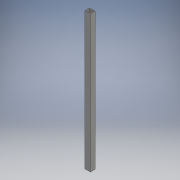
# Autodesk Inventor part: perfil aluminio
Saved by Autodesk Inventor 2016 (Build 200138000, 138)
## iProperties
Created: 2016-06-24
Part Number: perfil aluminio
Material: Generic
Document SubType Name: Modeling
Designer: Admin
Density: 1 g/cm^3
Appearance: Default
Author: Admin
Autodesk Inventor part; units mm, degrees
ref_plane "YZ Plane" through (0, 0, 0) normal (1, 0, 0) x (0, 1, 0)
ref_plane "XZ Plane" through (0, 0, 0) normal (0, 1, 0) x (-1, 0, 0)
ref_plane "XY Plane" through (0, 0, 0) normal (0, 0, 1) x (1, 0, 0)
sketch "Sketch1" plane through (0, 0, 0) normal (0, 0, 1) x (1, 0, 0)
  line L0 (0, 0) -> (12, 0)
  line L1 (12, 0) -> (12, 10)
  line L2 (12, 10) -> (0, 10)
  line L3 (0, 10) -> (0, 0)
  dimension "d0" = 12
  dimension "d1" = 10
  constraints: 8 end point, 2 parallel, 1 horizontal, 1 perpendicular
  measures "d0" distance of L2.end L1.end
  measures "d1" distance of L1.end L0.end
extrude "Extrusion1" add sketch "Sketch1" along normal blind 300
sketch "Sketch3" plane through (0, 0, 300) normal (0, 0, 1) x (1, 0, 0)
  line L0 (12, 10) -> (0, 10) projected
  line L1 (1, 1) -> (11, 1)
  line L2 (11, 1) -> (11, 9)
  line L3 (11, 9) -> (1, 9)
  line L4 (1, 9) -> (1, 1)
  line L5 (11, 1) -> (1, 9) construction
  point P0 (0, 0)
  point P1 (6, 5)
  constraints: 10 end point, 2 parallel, 1 horizontal, 1 midpoint, 1 perpendicular
extrude "Extrusion3" cut sketch "Sketch3" against normal through all
body "Solid1"
